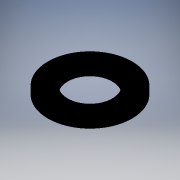
# Autodesk Inventor part: 11-6040
Saved by Autodesk Inventor 2017.3 (Build 213256000, 256)
## iProperties
Part Number: 11-6040
Material: Generic
Catalog Web Link: www.cadenas.de
Description: 11-6039, 11-6040, 11-6041, 11-6042-Flat Washers, Black Zinc
Vendor: 8020
Document SubType Name: Modeling
Designer: partserver
Manufacturer: 8020
Mass: 0.0508302 g
Surface Area: 1.56216 cm^2
Volume: 0.0508302 cm^3
Density: 1 g/cm^3
Appearance: PSOLRGB-0-0-0
Category: PARTsolutions
Company: 8020
Title: 11-6040
Author: Cadenas PARTsolutions
Comments: Flat Washers, Black Zinc
PSOL_IDENT_0: {$CADENAS_DATA\23d-libs\8020\metric\fastening_options\11_6039.prj},182 {VTYP=3D},{NB=11-6040},{LINA=
PSOL_IDENT_1: 11-6040},{NN=11-6039, 11-6040, 11-6041, 11-6042},{DATE=31.07.2020 09:21:25},{GEOMDATE=05.10.2017 15:
PSOL_IDENT_2: 57:59},{VERSION=},{LINEID=30},{WBVAR=},{WBNUMERIC=}  {NB=11-6040},{LINA=11-6040},{KT=DUMMY},{PN=11-6
PSOL_IDENT_3: 040},{FIN=Black-Coated},{SIZE=M5},{HS=5.30},{T=0.90},{W=.0007},{OD=10}
NB: 11-6040
NN: 11-6039, 11-6040, 11-6041, 11-6042
NT: Flat Washers, Black Zinc
NBSYN: $PN.
LINA: 11-6040
CATALOG: 80/20
PN: 11-6040
FIN: Black-Coated
SIZE: M5
HS: 5.3
T: 0.9
W: .0007
SUPPLIER: 8020
ARTICLENO: 11-6040
BOMINFO: 11-6040
CREATOR: CADENAS GmbH
Autodesk Inventor part; units mm, degrees
sketch "Sketch_1" plane through (0, 0, 0) normal (0, 0, 1) x (1, 0, 0)
  circle A0 centre (0, 0) radius 5
  circle A1 centre (0, 0) radius 2.65
  constraints: 2 centre point
extrude "Extrusion1" add sketch "Sketch_1" along normal mid plane 0.9
ref_plane "to_bolt_XY" through (0, 0, 0.45) normal (0, 0, 1) x (1, 0, 0)
ref_plane "to_bolt_YZ" through (0, 0, 0.45) normal (1, 0, 0) x (0, 1, 0)
ref_plane "to_bolt_ZX" through (0, 0, 0.45) normal (0, 1, 0) x (0, 0, 1)
ref_plane "to_profile_XY" through (0, 0, -0.45) normal (0, 0, 1) x (1, 0, 0)
ref_plane "to_profile_YZ" through (0, 0, -0.45) normal (1, 0, 0) x (0, 1, 0)
ref_plane "to_profile_ZX" through (0, 0, -0.45) normal (0, 1, 0) x (0, 0, 1)
ref_plane "washer_XY" through (0, 0, 0) normal (0, 0, 1) x (1, 0, 0)
ref_plane "washer_YZ" through (0, 0, 0) normal (1, 0, 0) x (0, 1, 0)
ref_plane "washer_ZX" through (0, 0, 0) normal (0, 1, 0) x (0, 0, 1)
body "Solid1"
